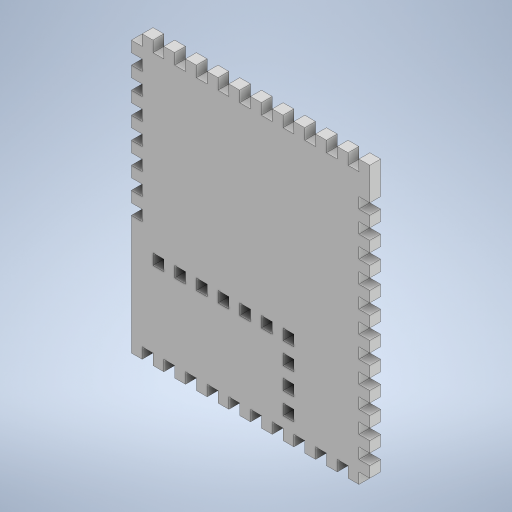
# Autodesk Inventor part: topsidesketch
Saved by Autodesk Inventor 2024 (Build 280153000, 153)
## iProperties
Created: 2024-04-15
Part Number: topsidesketch
Material: Generic
Document SubType Name: Modeling
Designer: srika
Density: 1 g/cm^3
Appearance: Default
Author: srika
Autodesk Inventor part; units mm, degrees
ref_plane "YZ Plane" through (0, 0, 0) normal (1, 0, 0) x (0, 1, 0)
ref_plane "XZ Plane" through (0, 0, 0) normal (0, 1, 0) x (-1, 0, 0)
ref_plane "XY Plane" through (0, 0, 0) normal (0, 0, 1) x (1, 0, 0)
sketch "Sketch1" plane through (0, 0, 0) normal (0, 0, 1) x (1, 0, 0)
  line L0 (5, 5) -> (105, 5)
  line L1 (105, 45) -> (105, 125)
  line L2 (105, 125) -> (5, 125)
  line L3 (5, 85) -> (5, 5)
  line L4 (0, 0) -> (5, 0)
  line L5 (5, 0) -> (5, 5)
  line L6 (5, 5) -> (0, 5)
  line L7 (0, 5) -> (0, 0)
  line L8 (105, 125) -> (110, 125)
  line L9 (110, 125) -> (110, 130)
  line L10 (110, 130) -> (105, 130)
  line L11 (105, 130) -> (105, 125)
  line L12 (5, 125) -> (5, 85)
  line L13 (105, 45) -> (105, 5)
  line L14 (5, 15) -> (0, 15)
  line L15 (0, 10) -> (5, 10)
  line L16 (0, 15) -> (0, 10)
  line L17 (5, 10) -> (5, 15)
  line L18 (5, 25) -> (0, 25)
  line L19 (0, 20) -> (5, 20)
  line L20 (0, 25) -> (0, 20)
  line L21 (5, 20) -> (5, 25)
  line L22 (5, 35) -> (0, 35)
  line L23 (0, 30) -> (5, 30)
  line L24 (0, 35) -> (0, 30)
  line L25 (5, 30) -> (5, 35)
  line L26 (5, 45) -> (0, 45)
  line L27 (0, 40) -> (5, 40)
  line L28 (0, 45) -> (0, 40)
  line L29 (5, 40) -> (5, 45)
  line L30 (5, 55) -> (0, 55)
  line L31 (0, 50) -> (5, 50)
  line L32 (0, 55) -> (0, 50)
  line L33 (5, 50) -> (5, 55)
  line L34 (5, 65) -> (0, 65)
  line L35 (0, 60) -> (5, 60)
  line L36 (0, 65) -> (0, 60)
  line L37 (5, 60) -> (5, 65)
  line L38 (5, 75) -> (0, 75)
  line L39 (0, 70) -> (5, 70)
  line L40 (0, 75) -> (0, 70)
  line L41 (5, 70) -> (5, 75)
  line L42 (5, 85) -> (0, 85)
  line L43 (0, 80) -> (5, 80)
  line L44 (0, 85) -> (0, 80)
  line L45 (5, 80) -> (5, 85)
  line L46 (5, 95) -> (0, 95)
  line L47 (0, 90) -> (5, 90)
  line L48 (0, 95) -> (0, 90)
  line L49 (5, 90) -> (5, 95)
  line L50 (5, 105) -> (0, 105)
  line L51 (0, 100) -> (5, 100)
  line L52 (0, 105) -> (0, 100)
  line L53 (5, 100) -> (5, 105)
  line L54 (5, 115) -> (0, 115)
  line L55 (0, 110) -> (5, 110)
  line L56 (0, 115) -> (0, 110)
  line L57 (5, 110) -> (5, 115)
  line L58 (5, 125) -> (0, 125)
  line L59 (0, 120) -> (5, 120)
  line L60 (0, 125) -> (0, 120)
  line L61 (5, 120) -> (5, 125)
  line L62 (10, 0) -> (15, 0)
  line L63 (15, 0) -> (15, 5)
  line L64 (15, 5) -> (10, 5)
  line L65 (10, 5) -> (10, 0)
  line L66 (20, 0) -> (25, 0)
  line L67 (25, 0) -> (25, 5)
  line L68 (25, 5) -> (20, 5)
  line L69 (20, 5) -> (20, 0)
  line L70 (30, 0) -> (35, 0)
  line L71 (35, 0) -> (35, 5)
  line L72 (35, 5) -> (30, 5)
  line L73 (30, 5) -> (30, 0)
  line L74 (40, 0) -> (45, 0)
  line L75 (45, 0) -> (45, 5)
  line L76 (45, 5) -> (40, 5)
  line L77 (40, 5) -> (40, 0)
  line L78 (50, 0) -> (55, 0)
  line L79 (55, 0) -> (55, 5)
  line L80 (55, 5) -> (50, 5)
  line L81 (50, 5) -> (50, 0)
  line L82 (60, 0) -> (65, 0)
  line L83 (65, 0) -> (65, 5)
  line L84 (65, 5) -> (60, 5)
  line L85 (60, 5) -> (60, 0)
  line L86 (70, 0) -> (75, 0)
  line L87 (75, 0) -> (75, 5)
  line L88 (75, 5) -> (70, 5)
  line L89 (70, 5) -> (70, 0)
  line L90 (80, 0) -> (85, 0)
  line L91 (85, 0) -> (85, 5)
  line L92 (85, 5) -> (80, 5)
  line L93 (80, 5) -> (80, 0)
  line L94 (90, 0) -> (95, 0)
  line L95 (95, 0) -> (95, 5)
  line L96 (95, 5) -> (90, 5)
  line L97 (90, 5) -> (90, 0)
  line L98 (100, 0) -> (105, 0)
  line L99 (105, 0) -> (105, 5)
  line L100 (105, 5) -> (100, 5)
  line L101 (100, 5) -> (100, 0)
  line L102 (105, 120) -> (105, 115)
  line L103 (110, 120) -> (105, 120)
  line L104 (110, 115) -> (110, 120)
  line L105 (105, 115) -> (110, 115)
  line L106 (105, 110) -> (105, 105)
  line L107 (110, 110) -> (105, 110)
  line L108 (110, 105) -> (110, 110)
  line L109 (105, 105) -> (110, 105)
  line L110 (105, 100) -> (105, 95)
  line L111 (110, 100) -> (105, 100)
  line L112 (110, 95) -> (110, 100)
  line L113 (105, 95) -> (110, 95)
  line L114 (105, 90) -> (105, 85)
  line L115 (110, 90) -> (105, 90)
  line L116 (110, 85) -> (110, 90)
  line L117 (105, 85) -> (110, 85)
  line L118 (105, 80) -> (105, 75)
  line L119 (110, 80) -> (105, 80)
  line L120 (110, 75) -> (110, 80)
  line L121 (105, 75) -> (110, 75)
  line L122 (105, 70) -> (105, 65)
  line L123 (110, 70) -> (105, 70)
  line L124 (110, 65) -> (110, 70)
  line L125 (105, 65) -> (110, 65)
  line L126 (105, 60) -> (105, 55)
  line L127 (110, 60) -> (105, 60)
  line L128 (110, 55) -> (110, 60)
  line L129 (105, 55) -> (110, 55)
  line L130 (105, 50) -> (105, 45)
  line L131 (110, 50) -> (105, 50)
  line L132 (110, 45) -> (110, 50)
  line L133 (105, 45) -> (110, 45)
  line L134 (105, 40) -> (105, 35)
  line L135 (110, 40) -> (105, 40)
  line L136 (110, 35) -> (110, 40)
  line L137 (105, 35) -> (110, 35)
  line L138 (105, 30) -> (105, 25)
  line L139 (110, 30) -> (105, 30)
  line L140 (110, 25) -> (110, 30)
  line L141 (105, 25) -> (110, 25)
  line L142 (105, 20) -> (105, 15)
  line L143 (110, 20) -> (105, 20)
  line L144 (110, 15) -> (110, 20)
  line L145 (105, 15) -> (110, 15)
  line L146 (105, 10) -> (105, 5)
  line L147 (110, 10) -> (105, 10)
  line L148 (110, 5) -> (110, 10)
  line L149 (105, 5) -> (110, 5)
  line L150 (95, 130) -> (95, 125)
  line L151 (100, 130) -> (95, 130)
  line L152 (100, 125) -> (100, 130)
  line L153 (95, 125) -> (100, 125)
  line L154 (85, 130) -> (85, 125)
  line L155 (90, 130) -> (85, 130)
  line L156 (90, 125) -> (90, 130)
  line L157 (85, 125) -> (90, 125)
  line L158 (75, 130) -> (75, 125)
  line L159 (80, 130) -> (75, 130)
  line L160 (80, 125) -> (80, 130)
  line L161 (75, 125) -> (80, 125)
  line L162 (65, 130) -> (65, 125)
  line L163 (70, 130) -> (65, 130)
  line L164 (70, 125) -> (70, 130)
  line L165 (65, 125) -> (70, 125)
  line L166 (55, 130) -> (55, 125)
  line L167 (60, 130) -> (55, 130)
  line L168 (60, 125) -> (60, 130)
  line L169 (55, 125) -> (60, 125)
  line L170 (45, 130) -> (45, 125)
  line L171 (50, 130) -> (45, 130)
  line L172 (50, 125) -> (50, 130)
  line L173 (45, 125) -> (50, 125)
  line L174 (35, 130) -> (35, 125)
  line L175 (40, 130) -> (35, 130)
  line L176 (40, 125) -> (40, 130)
  line L177 (35, 125) -> (40, 125)
  line L178 (25, 130) -> (25, 125)
  line L179 (30, 130) -> (25, 130)
  line L180 (30, 125) -> (30, 130)
  line L181 (25, 125) -> (30, 125)
  line L182 (15, 130) -> (15, 125)
  line L183 (20, 130) -> (15, 130)
  line L184 (20, 125) -> (20, 130)
  line L185 (15, 125) -> (20, 125)
  line L186 (5, 130) -> (5, 125)
  line L187 (10, 130) -> (5, 130)
  line L188 (10, 125) -> (10, 130)
  line L189 (5, 125) -> (10, 125)
  line L190 (105, 125) -> (110, 125)
  line L191 (110, 125) -> (110, 110)
  line L192 (110, 110) -> (105, 110)
  line L193 (105, 110) -> (105, 125)
  line L194 (5, 5) -> (0, 5)
  line L195 (0, 5) -> (0, 50)
  line L196 (0, 50) -> (5, 50)
  line L197 (5, 50) -> (5, 5)
  line L198 (0, 5) -> (70, 5)
  line L199 (70, 5) -> (70, 40)
  line L200 (70, 40) -> (0, 40)
  line L201 (0, 40) -> (0, 5)
  line L202 (10, 45) -> (15, 45)
  line L203 (15, 45) -> (15, 40)
  line L204 (15, 40) -> (10, 40)
  line L205 (10, 40) -> (10, 45)
  line L206 (20, 40) -> (20, 45)
  line L207 (20, 45) -> (25, 45)
  line L208 (25, 45) -> (25, 40)
  line L209 (30, 40) -> (30, 45)
  line L210 (30, 45) -> (35, 45)
  line L211 (35, 45) -> (35, 40)
  line L212 (40, 40) -> (40, 45)
  line L213 (40, 45) -> (45, 45)
  line L214 (45, 45) -> (45, 40)
  line L215 (50, 40) -> (50, 45)
  line L216 (50, 45) -> (55, 45)
  line L217 (55, 45) -> (55, 40)
  line L218 (60, 40) -> (60, 45)
  line L219 (60, 45) -> (65, 45)
  line L220 (65, 45) -> (65, 40)
  line L221 (70, 10) -> (75, 10)
  line L222 (75, 10) -> (75, 15)
  line L223 (75, 15) -> (70, 15)
  line L224 (70, 15) -> (70, 10)
  line L225 (75, 20) -> (75, 25)
  line L226 (75, 25) -> (70, 25)
  line L227 (70, 20) -> (75, 20)
  line L228 (75, 30) -> (75, 35)
  line L229 (75, 35) -> (70, 35)
  line L230 (70, 30) -> (75, 30)
  line L231 (75, 40) -> (75, 45)
  line L232 (75, 45) -> (70, 45)
  line L233 (70, 40) -> (75, 40)
  line L234 (70, 45) -> (70, 40)
  point P0 (7.75, 7)
  point P1 (7.75, 17)
  point P2 (7.75, 27)
  point P3 (7.75, 37)
  point P4 (7.75, 47)
  point P5 (7.75, 57)
  point P6 (7.75, 67)
  point P7 (7.75, 77)
  point P8 (7.75, 87)
  point P9 (7.75, 97)
  point P10 (7.75, 107)
  point P11 (7.75, 117)
  point P12 (7.75, 127)
  point P13 (105, 115)
  point P14 (105, 105)
  point P15 (105, 95)
  point P16 (105, 85)
  point P17 (105, 75)
  point P18 (105, 65)
  point P19 (105, 55)
  point P20 (105, 35)
  point P21 (105, 25)
  point P22 (105, 15)
  point P23 (95, 125)
  point P24 (85, 125)
  point P25 (75, 125)
  point P26 (65, 125)
  point P27 (55, 125)
  point P28 (45, 125)
  point P29 (35, 125)
  point P30 (25, 125)
  point P31 (15, 125)
  point P32 (5, 125)
  dimension "d0" = 100
  dimension "d1" = 80
  dimension "d16" = 5
  dimension "d17" = 5
  dimension "d39" = 10
  dimension "d46" = 10
  dimension "d53" = 10
  dimension "d60" = 10
  dimension "d69" = 10
  dimension "d76" = 10
  dimension "d81" = 65
  dimension "d82" = 35
  constraints: 464 end point, 90 horizontal alignment, 78 parallel, 64 collinear, 60 vertical alignment, 8 horizontal, 7 perpendicular, 6 vertical, 2 point on line, 173 other
  measures "d0" distance of L12.start L8.start
  measures "d1" distance of L190.start L13.start
  measures "d16" distance of L10.end L9.end
  measures "d17" distance of L9.end L8.end
  measures "d39" distance of L3.end L14.start
  measures "d46" distance of L3.end L63.end
  measures "d53" distance of L8.start L102.end
  measures "d60" distance of L10.end L150.start
  measures "d69" distance of L202.start L206.end
  measures "d76" distance of L222.end L225.end
  measures "d81" distance of L199.end L27.end
  measures "d82" distance of L198.end L199.end
extrude "Extrusion1" add sketch "Sketch1" along normal blind 5 contours L3 L200 L199 L0 | L6 L195 L15 L3 | L5 L4 L7 L6 | L0 L63 L62 L65 | L15 L16 L14 L3 | L14 L195 L19 L3 | L0 L67 L66 L69 | L19 L20 L18 L3 | L18 L195 L23 L3 | L0 L71 L70 L73 | L23 L24 L22 L3 | L22 L195 L27 L3 | L0 L75 L74 L77 | L27 L28 L26 L3 | L3 L12 L2 L1 L13 L0 L199 L221 L222 L223 L227 L225 L226 L230 L228 L229 L200 L220 L219 L218 L217 L216 L215 L214 L213 L212 L211 L210 L209 L208 L207 L206 L203 L202 L205 | L26 L195 L31 L3 | L0 L79 L78 L81 | L31 L32 L30 L3 | L0 L83 L82 L85 | L35 L36 L34 L3 | L0 L87 L86 L89 | L39 L40 L38 L3 | L0 L91 L90 L93 | L43 L44 L42 L3 | L0 L95 L94 L97 | L47 L48 L46 L12 | L0 L99 L98 L101 | L51 L52 L50 L12 | L13 L147 L148 L149 | L55 L56 L54 L12 | L13 L143 L144 L145 | L59 L60 L58 L12 | L13 L139 L140 L141 | L186 L187 L188 L2 | L13 L135 L136 L137 | L182 L183 L184 L2 | L1 L131 L132 L133 | L178 L179 L180 L2 | L1 L127 L128 L129 | L174 L175 L176 L2 | L1 L123 L124 L125 | L170 L171 L172 L2 | L1 L119 L120 L121 | L166 L167 L168 L2 | L1 L115 L116 L117 | L162 L163 L164 L2 | L1 L111 L112 L113 | L158 L159 L160 L2 | L1 L107 L108 L109 | L154 L155 L156 L2 | L1 L103 L104 L105 | L150 L151 L152 L2 | L1 L8 L191 L103 | L11 L10 L9 L8
body "Solid1"
